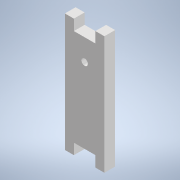
# Autodesk Inventor part: Z-Kettenhalter
Saved by Autodesk Inventor 2022 (Build 260153000, 153)
## iProperties
Created: 2021-04-27
Part Number: Z-Kettenhalter
Material: Generic
Document SubType Name: Modeling
Designer: Fabijan_Sven
Density: 1 g/cm^3
Appearance: Default
Author: Fabijan_Sven
Autodesk Inventor part; units mm, degrees
ref_plane "YZ Plane" through (0, 0, 0) normal (1, 0, 0) x (0, 1, 0)
ref_plane "XZ Plane" through (0, 0, 0) normal (0, 1, 0) x (-1, 0, 0)
ref_plane "XY Plane" through (0, 0, 0) normal (0, 0, 1) x (1, 0, 0)
sketch "Sketch1" plane through (0, 0, 0) normal (0, 0, 1) x (1, 0, 0)
  line L0 (0, 0) -> (18, 0) construction
  line L1 (18, -55) -> (0, -55) construction
  line L2 (-0.2, 0) -> (4, 0)
  line L3 (18.2, 0) -> (18.2, -55)
  line L4 (18.2, -55) -> (14, -55)
  line L5 (-0.2, -55) -> (-0.2, 0)
  line L6 (14, 0) -> (14, -5)
  line L7 (14, -5) -> (4, -5)
  line L8 (4, -5) -> (4, 0)
  line L9 (14, 0) -> (18.2, 0)
  line L10 (14, -55) -> (14, -49.9766)
  line L11 (14, -49.9766) -> (4, -49.9766)
  line L12 (4, -49.9766) -> (4, -55)
  line L13 (4, -55) -> (-0.2, -55)
  point P0 (1, -55)
  point P1 (16.8146, 0)
  point P2 (4, -2.5)
  point P3 (4, -52.4883)
  point P4 (14, -52.4883)
  point P5 (14, -2.5)
  dimension "d33" = 18.4
  dimension "d34" = 0.2
  dimension "d35" = 4.2
  dimension "d36" = 4.2
  dimension "d37" = 5
  dimension "d38" = 0
  dimension "d39" = 5.0234
  dimension "d40" = 0
  constraints: 24 end point, 7 parallel, 4 midpoint, 2 horizontal, 2 perpendicular, 2 point on line, 2 vertical alignment, 1 vertical
  measures "d33" distance between parallel lines of L3 L5
  measures "d34" distance of L2.start L0.start
  measures "d35" distance between parallel lines of L8 L5
  measures "d36" distance between parallel lines of L3 L6
  measures "d37" distance between parallel lines of L7 L0
  measures "d38" distance between parallel lines of L2 L9
  measures "d39" distance between parallel lines of L1 L11
  measures "d40" distance between parallel lines of L1 L13
extrude "Extrusion1" add sketch "Sketch1" along normal blind 5
sketch "Sketch3" plane through (0, 0, 5) normal (0, 0, 1) x (1, 0, 0)
  line L0 (-0.2, 0) -> (-0.2, -55) projected
  circle A0 centre (9, -15) radius 1.5
  line L1 (4, 0) -> (-0.2, 0) projected
  point P0 (0, 0)
  point P1 (1, -55)
  dimension "d21" = 3
  dimension "d25" = 9.2
  dimension "d41" = 15
  constraints: 1 centre point, 1 other
  measures "d21" diameter of A0
  measures "d41" distance from line of A0.centre L1
hole "Hole2" at (9, -15, 5) direction (0, 0, -1) diameter 3 depth 8 tip angle 118
equation "\"d26\" = d21"
body "Solid1"
